Autodesk Inventor part; units mm, degrees
(part 2 of 2)
  spline S289 degree 2 poles (-17.6351, 28.7102) (-17.8218, 28.9306) (-18.2282, 29.1) (-18.7854, 29.0036) (-19.0563, 28.8252) knots 0 0 0 1 2 3 3 3
  spline S290 degree 2 poles (-19.0563, 28.8252) (-19.2958, 28.6675) (-19.572, 28.2811) (-19.5869, 27.9141) (-19.4898, 27.7665) knots 0 0 0 1 2 3 3 3
  spline S291 degree 2 poles (-19.4898, 27.7665) (-19.391, 27.6166) (-19.0728, 27.5071) (-18.8226, 27.5643) knots 0 0 0 1 2 2 2
  spline S292 degree 2 poles (-18.8226, 27.5643) (-18.6609, 27.5979) (-17.6442, 27.9656) (-17.4055, 27.9875) knots 0 0 0 1 2 2 2
  spline S293 degree 2 poles (-17.4055, 27.9875) (-17.1001, 28.0187) (-16.645, 27.812) (-16.5017, 27.5943) knots 0 0 0 1 2 2 2
  spline S294 degree 2 poles (-16.5017, 27.5943) (-16.3424, 27.3524) (-16.3418, 26.7563) (-16.7234, 26.193) (-17.0451, 25.9812) knots 0 0 0 1 2 3 3 3
  spline S295 degree 2 poles (-17.0451, 25.9812) (-17.3983, 25.7486) (-18.0875, 25.6209) (-18.6717, 25.8708) (-18.8645, 26.1427) knots 0 0 0 1 2 3 3 3
  line L241 (-18.8645, 26.1427) -> (-18.4836, 26.4385)
  spline S296 degree 2 poles (-18.4836, 26.4385) (-18.2531, 26.1568) (-17.6735, 26.0981) (-17.3058, 26.3401) knots 0 0 0 1 2 2 2
  spline S297 degree 2 poles (-17.3058, 26.3401) (-16.9235, 26.5918) (-16.7575, 27.1034) (-16.8865, 27.2993) knots 0 0 0 1 2 2 2
  spline S298 degree 2 poles (-16.8865, 27.2993) (-16.9996, 27.4711) (-17.1963, 27.5011) knots 0 0 0 1 1 1
  spline S299 degree 2 poles (-17.1963, 27.5011) (-17.3913, 27.5287) (-18.5723, 27.0841) (-18.8208, 27.0453) knots 0 0 0 1 2 2 2
  spline S300 degree 2 poles (-18.8208, 27.0453) (-19.181, 26.992) (-19.7027, 27.2103) (-19.8699, 27.4643) knots 0 0 0 1 2 2 2
  spline S301 degree 2 poles (-19.8699, 27.4643) (-20.0371, 27.7183) (-20.0415, 28.3569) (-19.6612, 28.9645) (-19.3226, 29.1874) knots 0 0 0 1 2 3 3 3
  spline S302 degree 2 poles (-19.3226, 29.1874) (-18.8895, 29.4725) (-18.1433, 29.6032) (-17.4806, 29.3182) (-17.2607, 29.0053) knots 0 0 0 1 2 3 3 3
  spline S303 degree 2 poles (-22.1485, 26.5919) (-22.0826, 26.9267) (-21.8218, 27.3655) (-21.607, 27.5375) knots 0 0 0 1 2 2 2
  spline S304 degree 2 poles (-21.607, 27.5375) (-21.252, 27.8217) (-20.5952, 27.7799) (-20.3798, 27.5108) knots 0 0 0 1 2 2 2
  spline S305 degree 2 poles (-20.3798, 27.5108) (-20.2531, 27.3525) (-20.1896, 26.9767) (-20.2935, 26.6338) (-20.4097, 26.4777) knots 0 0 0 1 2 3 3 3
  spline S306 degree 2 poles (-20.4097, 26.4777) (-20.4924, 26.3632) (-20.6878, 26.1623) knots 0 0 0 1 1 1
  spline S307 degree 2 poles (-20.6878, 26.1623) (-21.087, 25.7573) (-21.2371, 25.5184) knots 0 0 0 1 1 1
  spline S308 degree 2 poles (-21.2371, 25.5184) (-21.1797, 25.442) (-21.1634, 25.4217) knots 0 0 0 1 1 1
  spline S309 degree 2 poles (-21.1634, 25.4217) (-20.9842, 25.1978) (-20.8077, 25.1906) knots 0 0 0 1 1 1
  spline S310 degree 2 poles (-20.8077, 25.1906) (-20.5703, 25.1767) (-20.2944, 25.3975) knots 0 0 0 1 1 1
  spline S311 degree 2 poles (-20.2944, 25.3975) (-20.0389, 25.6021) (-19.9396, 25.9785) (-20.0636, 26.2539) knots 0 0 0 1 2 2 2
  line L242 (-20.0636, 26.2539) -> (-19.6683, 26.4924)
  spline S312 degree 2 poles (-19.6683, 26.4924) (-19.533, 26.226) (-19.5306, 25.7642) (-19.8298, 25.276) (-20.1057, 25.0552) knots 0 0 0 1 2 3 3 3
  spline S313 degree 2 poles (-20.1057, 25.0552) (-20.3815, 24.8344) (-20.8284, 24.6881) (-21.1486, 24.7545) (-21.2998, 24.8784) knots 0 0 0 1 2 3 3 3
  spline S314 degree 2 poles (-21.2998, 24.8784) (-21.3939, 24.9588) (-21.5876, 25.2008) knots 0 0 0 1 1 1
  line L243 (-21.5876, 25.2008) -> (-21.9768, 25.6869)
  spline S315 degree 2 poles (-21.9768, 25.6869) (-22.3822, 26.1933) (-22.6451, 26.4244) (-22.8125, 26.4944) knots 0 0 0 1 2 2 2
  line L244 (-22.8125, 26.4944) -> (-22.4327, 26.7985)
  spline S316 degree 2 poles (-22.4327, 26.7985) (-22.2856, 26.7307) (-22.1485, 26.5919) knots 0 0 0 1 1 1
  spline S317 degree 2 poles (-21.4675, 25.8015) (-21.3337, 26.0422) (-20.9832, 26.4155) knots 0 0 0 1 1 1
  spline S318 degree 2 poles (-20.9832, 26.4155) (-20.7825, 26.6282) (-20.6623, 26.858) (-20.6854, 27.0955) (-20.7614, 27.1904) knots 0 0 0 1 2 3 3 3
  spline S319 degree 2 poles (-20.7614, 27.1904) (-20.8773, 27.3351) (-21.2523, 27.354) (-21.4648, 27.1838) knots 0 0 0 1 2 2 2
  spline S320 degree 2 poles (-21.4648, 27.1838) (-21.6751, 27.0155) (-21.8563, 26.5699) (-21.8047, 26.3478) knots 0 0 0 1 2 2 2
  spline S321 degree 2 poles (-21.8047, 26.3478) (-21.7639, 26.1764) (-21.572, 25.9367) knots 0 0 0 1 1 1
  line L245 (-21.572, 25.9367) -> (-21.4675, 25.8015)
  line L246 (-23.2232, 26.1065) -> (-20.6773, 23.2854)
  line L247 (-20.6773, 23.2854) -> (-21.0235, 22.973)
  line L248 (-21.0235, 22.973) -> (-23.5694, 25.7941)
  line L249 (-23.5694, 25.7941) -> (-23.2232, 26.1065)
  line L250 (-23.9341, 25.4845) -> (-23.6648, 25.2172)
  line L251 (-23.6648, 25.2172) -> (-23.4708, 22.5596)
  spline S322 degree 2 poles (-23.4708, 22.5596) (-23.2709, 22.7815) (-23.1097, 22.9439) knots 0 0 0 1 1 1
  line L252 (-23.1097, 22.9439) -> (-22.322, 23.7373)
  line L253 (-22.322, 23.7373) -> (-22.0528, 23.47)
  line L254 (-22.0528, 23.47) -> (-23.6362, 21.8749)
  line L255 (-23.6362, 21.8749) -> (-23.8562, 22.0933)
  line L256 (-23.8562, 22.0933) -> (-24.0447, 24.3823)
  line L257 (-24.0447, 24.3823) -> (-24.0688, 24.8102)
  spline S323 degree 2 poles (-24.0688, 24.8102) (-24.2748, 24.5699) (-24.4687, 24.3746) knots 0 0 0 1 1 1
  line L258 (-24.4687, 24.3746) -> (-25.3645, 23.4722)
  line L259 (-25.3645, 23.4722) -> (-25.6502, 23.7559)
  line L260 (-25.6502, 23.7559) -> (-23.9341, 25.4845)
  line L261 (-26.239, 23.0826) -> (-25.9605, 23.4122)
  line L262 (-25.9605, 23.4122) -> (-23.0579, 20.9597)
  line L263 (-23.0579, 20.9597) -> (-23.3588, 20.6035)
  line L264 (-23.3588, 20.6035) -> (-24.3942, 21.4783)
  spline S324 degree 2 poles (-24.3942, 21.4783) (-24.3017, 21.0134) (-24.597, 20.6638) knots 0 0 0 1 1 1
  spline S325 degree 2 poles (-24.597, 20.6638) (-24.7615, 20.4691) (-25.2121, 20.2545) (-25.6841, 20.2703) (-26.1889, 20.4807) (-26.4167, 20.6733) knots 0 0 0 1 2 3 4 4 4
  spline S326 degree 2 poles (-26.4167, 20.6733) (-26.9565, 21.1294) (-27.0949, 22.1639) (-26.7789, 22.5378) knots 0 0 0 1 2 2 2
  spline S327 degree 2 poles (-26.7789, 22.5378) (-26.4649, 22.9094) (-25.9757, 22.8601) knots 0 0 0 1 1 1
  line L265 (-25.9757, 22.8601) -> (-26.239, 23.0826)
  spline S328 degree 2 poles (-25.1667, 22.1841) (-25.545, 22.5038) (-25.8013, 22.5459) knots 0 0 0 1 1 1
  spline S329 degree 2 poles (-25.8013, 22.5459) (-26.2177, 22.6096) (-26.4607, 22.322) knots 0 0 0 1 1 1
  spline S330 degree 2 poles (-26.4607, 22.322) (-26.657, 22.0897) (-26.5378, 21.405) (-26.1374, 21.0667) knots 0 0 0 1 2 2 2
  spline S331 degree 2 poles (-26.1374, 21.0667) (-25.7237, 20.7171) (-25.0573, 20.7115) (-24.861, 20.9438) knots 0 0 0 1 2 2 2
  spline S332 degree 2 poles (-24.861, 20.9438) (-24.6648, 21.1761) (-24.784, 21.8607) (-25.1667, 22.1841) knots 0 0 0 1 2 2 2
  line L266 (-28.8863, 19.6683) -> (-28.5556, 19.4336)
  spline S333 degree 2 poles (-28.5556, 19.4336) (-28.7499, 19.9657) (-28.4314, 20.4145) knots 0 0 0 1 1 1
  spline S334 degree 2 poles (-28.4314, 20.4145) (-28.2906, 20.6129) (-27.8947, 20.8505) (-27.5443, 20.8539) (-27.3531, 20.768) knots 0 0 0 1 2 3 3 3
  spline S335 degree 2 poles (-27.3531, 20.768) (-27.2253, 20.7128) (-26.982, 20.5402) knots 0 0 0 1 1 1
  line L267 (-26.982, 20.5402) -> (-25.5907, 19.553)
  line L268 (-25.5907, 19.553) -> (-25.8606, 19.1727)
  line L269 (-25.8606, 19.1727) -> (-27.1054, 20.056)
  spline S336 degree 2 poles (-27.1054, 20.056) (-27.403, 20.2672) (-27.5237, 20.3173) knots 0 0 0 1 1 1
  spline S337 degree 2 poles (-27.5237, 20.3173) (-27.7, 20.3891) (-28.0344, 20.2783) (-28.1567, 20.1059) knots 0 0 0 1 2 2 2
  spline S338 degree 2 poles (-28.1567, 20.1059) (-28.2774, 19.9358) (-28.3155, 19.5118) (-28.102, 19.1721) (-27.8138, 18.9676) knots 0 0 0 1 2 3 3 3
  line L270 (-27.8138, 18.9676) -> (-26.6115, 18.1144)
  line L271 (-26.6115, 18.1144) -> (-26.8814, 17.7341)
  line L272 (-26.8814, 17.7341) -> (-29.1277, 19.3281)
  line L273 (-29.1277, 19.3281) -> (-28.8863, 19.6683)
  line L274 (-29.5122, 18.7116) -> (-27.1635, 17.2727)
  line L275 (-27.1635, 17.2727) -> (-27.3829, 16.9146)
  line L276 (-27.3829, 16.9146) -> (-27.7385, 17.1325)
  spline S339 degree 2 poles (-27.7385, 17.1325) (-27.5723, 16.8438) (-27.5565, 16.5148) (-27.6427, 16.3741) knots 0 0 0 1 2 2 2
  spline S340 degree 2 poles (-27.6427, 16.3741) (-27.7653, 16.174) (-28.0183, 16.0437) knots 0 0 0 1 1 1
  line L277 (-28.0183, 16.0437) -> (-28.304, 16.409)
  spline S341 degree 2 poles (-28.304, 16.409) (-28.1283, 16.5017) (-28.0391, 16.6474) knots 0 0 0 1 1 1
  spline S342 degree 2 poles (-28.0391, 16.6474) (-27.9589, 16.7783) (-27.9914, 17.0802) (-28.1024, 17.2093) knots 0 0 0 1 2 2 2
  spline S343 degree 2 poles (-28.1024, 17.2093) (-28.274, 17.4061) (-28.5259, 17.5605) knots 0 0 0 1 1 1
  line L278 (-28.5259, 17.5605) -> (-29.7558, 18.3139)
  line L279 (-29.7558, 18.3139) -> (-29.5122, 18.7116)
  line L280 (-30.5948, 17.3802) -> (-30.8647, 17.0082)
  spline S344 degree 2 poles (-30.8647, 17.0082) (-31.0654, 17.0806) (-31.2105, 17.0094) knots 0 0 0 1 1 1
  spline S345 degree 2 poles (-31.2105, 17.0094) (-31.4066, 16.9159) (-31.5463, 16.649) knots 0 0 0 1 1 1
  spline S346 degree 2 poles (-31.5463, 16.649) (-31.6953, 16.3641) (-31.6308, 15.9316) (-31.4525, 15.7663) knots 0 0 0 1 2 2 2
  spline S347 degree 2 poles (-31.4525, 15.7663) (-31.3429, 15.6697) (-30.9386, 15.4614) knots 0 0 0 1 1 1
  spline S348 degree 2 poles (-30.9386, 15.4614) (-31.1158, 15.8974) (-30.9036, 16.3029) knots 0 0 0 1 1 1
  spline S349 degree 2 poles (-30.9036, 16.3029) (-30.6404, 16.8058) (-29.6254, 16.9775) (-29.1173, 16.7115) knots 0 0 0 1 2 2 2
  spline S350 degree 2 poles (-29.1173, 16.7115) (-28.7683, 16.5289) (-28.3111, 15.966) (-28.2414, 15.3182) (-28.4107, 14.9949) knots 0 0 0 1 2 3 3 3
  spline S351 degree 2 poles (-28.4107, 14.9949) (-28.6363, 14.5638) (-29.1317, 14.4667) knots 0 0 0 1 1 1
  line L281 (-29.1317, 14.4667) -> (-28.8366, 14.3123)
  line L282 (-28.8366, 14.3123) -> (-29.0367, 13.9299)
  line L283 (-29.0367, 13.9299) -> (-31.1435, 15.0325)
  spline S352 degree 2 poles (-31.1435, 15.0325) (-31.7132, 15.3307) (-32.0696, 15.8114) (-32.081, 16.4581) (-31.8876, 16.8276) knots 0 0 0 1 2 3 3 3
  spline S353 degree 2 poles (-31.8876, 16.8276) (-31.6592, 17.2639) (-30.9859, 17.5947) (-30.5948, 17.3802) knots 0 0 0 1 2 2 2
  spline S354 degree 2 poles (-29.312, 16.2708) (-29.7919, 16.5219) (-30.4334, 16.3706) (-30.5825, 16.0857) knots 0 0 0 1 2 2 2
  spline S355 degree 2 poles (-30.5825, 16.0857) (-30.7315, 15.8009) (-30.4942, 15.1863) (-30.0246, 14.9405) knots 0 0 0 1 2 2 2
  spline S356 degree 2 poles (-30.0246, 14.9405) (-29.5755, 14.7055) (-28.9145, 14.863) (-28.7681, 15.1427) knots 0 0 0 1 2 2 2
  spline S357 degree 2 poles (-28.7681, 15.1427) (-28.623, 15.4198) (-28.8707, 16.0398) (-29.312, 16.2708) knots 0 0 0 1 2 2 2
  constraints: 2 other
extrude "Extrusion2" add sketch "Skizze2" along normal blind 1 contours S0 S1 S2 L0 S3 S4 S5 S6 L1 S7 S8 | L2 L3 L4 L5 L6 L7 L8 | L9 L10 L11 L12 | S19 S20 S21 L13 L14 S22 S23 S24 S25 S26 S27 S28 L15 L16 L17 L18 L19 S29 S30 S31 | L20 S32 S33 S34 S35 L21 L22 L23 S36 S37 S38 L24 L25 L26 L27 L28 S39 S40 S41 S42 S43 L29 L30 | L31 S44 S45 S46 S47 L32 L33 L34 S48 S49 S50 L35 L36 L37 L38 L39 S51 S52 S53 S54 S55 L40 L41 | S56 L42 L43 L44 L45 L46 L47 L48 L49 L50 L51 L52 S57 S58 S59 L53 L54 S60 | S61 S62 S63 S64 | S69 S70 S71 L55 L56 S72 S73 S74 S75 S76 S77 S78 L57 L58 L59 L60 L61 S79 S80 S81 | S82 S83 L62 L63 S84 S85 S86 S87 L64 S88 S89 S90 S91 S92 L65 L66 S93 S94 S95 S96 S97 L67 L68 L69 S98 S99 S100 | L70 L71 L72 L73 | S101 S102 S103 L74 L75 S104 S105 S106 S107 S108 S109 S110 L76 L77 L78 L79 L80 S111 S112 S113 | L81 S114 S115 S116 S117 L82 L83 L84 S118 S119 S120 L85 L86 L87 L88 L89 S121 S122 S123 S124 S125 L90 L91 | L92 S126 S127 S128 S129 L93 L94 L95 S130 S131 S132 L96 L97 L98 L99 L100 S133 S134 S135 S136 S137 L101 L102 | L103 L104 S138 S139 S140 L105 L106 L107 | S144 S145 S146 S147 S148 S149 S150 S151 S152 L111 S153 S154 S155 L112 S156 L113 S157 | L115 L116 L117 S163 S164 L118 S165 S166 S167 L119 L120 | L121 L122 L123 L124 | L125 L126 L127 L128 | L129 S168 S169 S170 S171 S172 S173 S174 S175 L130 S176 S177 S178 S179 S180 S181 S182 S183 | L131 L132 L133 L134 L135 L136 | S184 S185 S186 S187 S188 | L137 S193 S194 S195 S196 L138 L139 L140 L141 | L142 L143 L144 S201 S202 L145 S203 S204 S205 L146 L147 | S206 S207 S208 S209 S210 | L148 L149 L150 S215 S216 S217 L151 L152 L153 S218 S219 L154 L155 | L156 L157 S220 S221 L158 L159 L160 S222 S223 L161 | L162 L163 L164 S224 S225 S226 L165 L166 L167 S227 S228 L168 L169 | L170 L171 L172 L173 | L174 L175 L176 L177 | L178 L179 L180 S229 S230 L181 L182 L183 L184 | L185 S231 S232 S233 S234 S235 L186 S236 S237 | L188 L189 L190 S241 S242 L191 S243 S244 S245 L192 L193 | L194 S246 S247 S248 S249 S250 S251 S252 S253 L195 S254 S255 S256 S257 S258 S259 S260 S261 | L196 L197 L198 L199 | L200 L201 L202 L203 | L204 S262 S263 L205 L206 L207 L208 L209 L210 L211 L212 L213 L214 L215 S264 S265 | S266 S267 S268 S269 S270 S271 S272 S273 S274 L216 S275 S276 S277 L217 S278 L218 S279 | L220 L221 L222 L223 | L224 L225 L226 L227 | L228 S285 S286 L229 L230 L231 L232 L233 L234 L235 L236 L237 L238 L239 S287 S288 | L240 S289 S290 S291 S292 S293 S294 S295 L241 S296 S297 S298 S299 S300 S301 S302 | S303 S304 S305 S306 S307 S308 S309 S310 S311 L242 S312 S313 S314 L243 S315 L244 S316 | L246 L247 L248 L249 | L250 L251 S322 L252 L253 L254 L255 L256 L257 S323 L258 L259 L260 | L261 L262 L263 L264 S324 S325 S326 S327 L265 | L266 S333 S334 S335 L267 L268 L269 S336 S337 S338 L270 L271 L272 L273 | L274 L275 L276 S339 S340 L277 S341 S342 S343 L278 L279 | L280 S344 S345 S346 S347 S348 S349 S350 S351 L281 L282 L283 S352 S353
